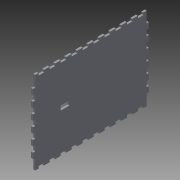
# Autodesk Inventor part: zijplaat
Saved by Autodesk Inventor 2015 (Build 190159000, 159)
## iProperties
Created: 2016-03-10
Part Number: zijplaat
Material: Generic
Document SubType Name: Modeling
Designer: david
Density: 1 g/cm^3
Appearance: Default
Author: david
Autodesk Inventor part; units mm, degrees
ref_plane "YZ Plane" through (0, 0, 0) normal (1, 0, 0) x (0, 1, 0)
ref_plane "XZ Plane" through (0, 0, 0) normal (0, 1, 0) x (-1, 0, 0)
ref_plane "XY Plane" through (0, 0, 0) normal (0, 0, 1) x (1, 0, 0)
sketch "Sketch1" plane through (0, 0, 0) normal (1, 0, 0) x (0, 1, 0)
  line L0 (0, 0) -> (210, 0)
  line L1 (210, 0) -> (210, 150)
  line L2 (210, 150) -> (0, 150)
  line L3 (0, 150) -> (0, 0)
  line L4 (66, 79) -> (50, 79)
  line L5 (50, 79) -> (50, 71)
  line L6 (50, 71) -> (66, 71)
  line L7 (66, 71) -> (66, 79)
  line L8 (0, 140) -> (4, 140)
  line L9 (4, 140) -> (4, 130)
  line L10 (4, 130) -> (0, 130)
  line L11 (0, 130) -> (0, 140)
  line L12 (0, 120) -> (4, 120)
  line L13 (4, 120) -> (4, 110)
  line L14 (4, 110) -> (0, 110)
  line L15 (0, 110) -> (0, 120)
  line L16 (0, 100) -> (4, 100)
  line L17 (4, 100) -> (4, 90)
  line L18 (4, 90) -> (0, 90)
  line L19 (0, 90) -> (0, 100)
  line L20 (0, 80) -> (4, 80)
  line L21 (4, 80) -> (4, 70)
  line L22 (4, 70) -> (0, 70)
  line L23 (0, 70) -> (0, 80)
  line L24 (0, 60) -> (4, 60)
  line L25 (4, 60) -> (4, 50)
  line L26 (4, 50) -> (0, 50)
  line L27 (0, 50) -> (0, 60)
  line L28 (0, 40) -> (4, 40)
  line L29 (4, 40) -> (4, 30)
  line L30 (4, 30) -> (0, 30)
  line L31 (0, 30) -> (0, 40)
  line L32 (0, 20) -> (4, 20)
  line L33 (4, 20) -> (4, 10)
  line L34 (4, 10) -> (0, 10)
  line L35 (0, 10) -> (0, 20)
  line L36 (10, 150) -> (20, 150)
  line L37 (20, 150) -> (20, 146)
  line L38 (20, 146) -> (10, 146)
  line L39 (10, 146) -> (10, 150)
  line L40 (30, 150) -> (40, 150)
  line L41 (40, 150) -> (40, 146)
  line L42 (40, 146) -> (30, 146)
  line L43 (30, 146) -> (30, 150)
  line L44 (50, 150) -> (60, 150)
  line L45 (60, 150) -> (60, 146)
  line L46 (60, 146) -> (50, 146)
  line L47 (50, 146) -> (50, 150)
  line L48 (70, 150) -> (80, 150)
  line L49 (80, 150) -> (80, 146)
  line L50 (80, 146) -> (70, 146)
  line L51 (70, 146) -> (70, 150)
  line L52 (90, 150) -> (100, 150)
  line L53 (100, 150) -> (100, 146)
  line L54 (100, 146) -> (90, 146)
  line L55 (90, 146) -> (90, 150)
  line L56 (110, 150) -> (120, 150)
  line L57 (120, 150) -> (120, 146)
  line L58 (120, 146) -> (110, 146)
  line L59 (110, 146) -> (110, 150)
  line L60 (130, 150) -> (140, 150)
  line L61 (140, 150) -> (140, 146)
  line L62 (140, 146) -> (130, 146)
  line L63 (130, 146) -> (130, 150)
  line L64 (150, 150) -> (160, 150)
  line L65 (160, 150) -> (160, 146)
  line L66 (160, 146) -> (150, 146)
  line L67 (150, 146) -> (150, 150)
  line L68 (170, 150) -> (180, 150)
  line L69 (180, 150) -> (180, 146)
  line L70 (180, 146) -> (170, 146)
  line L71 (170, 146) -> (170, 150)
  line L72 (190, 150) -> (200, 150)
  line L73 (200, 150) -> (200, 146)
  line L74 (200, 146) -> (190, 146)
  line L75 (190, 146) -> (190, 150)
  line L76 (0, 10) -> (4, 10)
  line L77 (4, 10) -> (4, 0)
  line L78 (4, 0) -> (0, 0)
  line L79 (0, 0) -> (0, 10)
  line L80 (0, 140) -> (4, 140)
  line L81 (4, 140) -> (4, 150)
  line L82 (4, 150) -> (0, 150)
  line L83 (0, 150) -> (0, 140)
  line L84 (10, 0) -> (20, 0)
  line L85 (20, 0) -> (20, 4)
  line L86 (20, 4) -> (10, 4)
  line L87 (10, 4) -> (10, 0)
  line L88 (30, 0) -> (40, 0)
  line L89 (40, 0) -> (40, 4)
  line L90 (40, 4) -> (30, 4)
  line L91 (30, 4) -> (30, 0)
  line L92 (50, 0) -> (60, 0)
  line L93 (60, 0) -> (60, 4)
  line L94 (60, 4) -> (50, 4)
  line L95 (50, 4) -> (50, 0)
  line L96 (70, 0) -> (80, 0)
  line L97 (80, 0) -> (80, 4)
  line L98 (80, 4) -> (70, 4)
  line L99 (70, 4) -> (70, 0)
  line L100 (90, 0) -> (100, 0)
  line L101 (100, 0) -> (100, 4)
  line L102 (100, 4) -> (90, 4)
  line L103 (90, 4) -> (90, 0)
  line L104 (110, 0) -> (120, 0)
  line L105 (120, 0) -> (120, 4)
  line L106 (120, 4) -> (110, 4)
  line L107 (110, 4) -> (110, 0)
  line L108 (130, 0) -> (140, 0)
  line L109 (140, 0) -> (140, 4)
  line L110 (140, 4) -> (130, 4)
  line L111 (130, 4) -> (130, 0)
  line L112 (150, 0) -> (160, 0)
  line L113 (160, 0) -> (160, 4)
  line L114 (160, 4) -> (150, 4)
  line L115 (150, 4) -> (150, 0)
  line L116 (170, 0) -> (180, 0)
  line L117 (180, 0) -> (180, 4)
  line L118 (180, 4) -> (170, 4)
  line L119 (170, 4) -> (170, 0)
  line L120 (190, 0) -> (200, 0)
  line L121 (200, 0) -> (200, 4)
  line L122 (200, 4) -> (190, 4)
  line L123 (190, 4) -> (190, 0)
  line L124 (210, 140) -> (206, 140)
  line L125 (206, 140) -> (206, 130)
  line L126 (206, 130) -> (210, 130)
  line L127 (210, 130) -> (210, 140)
  line L128 (210, 120) -> (206, 120)
  line L129 (206, 120) -> (206, 110)
  line L130 (206, 110) -> (210, 110)
  line L131 (210, 110) -> (210, 120)
  line L132 (210, 100) -> (206, 100)
  line L133 (206, 100) -> (206, 90)
  line L134 (206, 90) -> (210, 90)
  line L135 (210, 90) -> (210, 100)
  line L136 (210, 80) -> (206, 80)
  line L137 (206, 80) -> (206, 70)
  line L138 (206, 70) -> (210, 70)
  line L139 (210, 70) -> (210, 80)
  line L140 (210, 60) -> (206, 60)
  line L141 (206, 60) -> (206, 50)
  line L142 (206, 50) -> (210, 50)
  line L143 (210, 50) -> (210, 60)
  line L144 (210, 40) -> (206, 40)
  line L145 (206, 40) -> (206, 30)
  line L146 (206, 30) -> (210, 30)
  line L147 (210, 30) -> (210, 40)
  line L148 (210, 20) -> (206, 20)
  line L149 (206, 20) -> (206, 10)
  line L150 (206, 10) -> (210, 10)
  line L151 (210, 10) -> (210, 20)
  line L152 (206, 140) -> (206, 150)
  line L153 (206, 10) -> (206, 0)
  line L154 (206, 10) -> (210, 10)
  line L155 (210, 10) -> (210, 0)
  line L156 (210, 0) -> (206, 0)
  line L157 (206, 0) -> (206, 10)
  point P0 (0, 130)
  point P1 (0, 110)
  point P2 (0, 90)
  point P3 (0, 70)
  point P4 (0, 50)
  point P5 (0, 30)
  point P6 (24, 0)
  point P7 (44, 0)
  point P8 (64, 0)
  point P9 (84, 0)
  point P10 (104, 0)
  point P11 (124, 0)
  point P12 (144, 0)
  point P13 (164, 0)
  point P14 (184, 0)
  point P15 (210, 130)
  point P16 (210, 110)
  point P17 (210, 90)
  point P18 (210, 70)
  point P19 (210, 50)
  point P20 (210, 30)
  dimension "d0" = 150
  dimension "d1" = 210
  dimension "d2" = 8
  dimension "d3" = 16
  dimension "d4" = 71
  dimension "d5" = 50
  dimension "d6" = 4
  dimension "d7" = 10
  dimension "d8" = 10
  dimension "d11" = 20
  dimension "d16" = 4
  dimension "d17" = 10
  dimension "d18" = 10
  dimension "d21" = 20
  dimension "d26" = 4
  dimension "d27" = 10
  dimension "d30" = 20
  dimension "d35" = 4
  dimension "d36" = 10
  dimension "d37" = 10
  dimension "d40" = 20
  constraints: 316 end point, 18 parallel, 11 horizontal, 10 perpendicular, 10 point on line, 4 collinear, 2 vertical, 257 other
  measures "d0" distance of L2.end L0.start
  measures "d1" distance of L0.start L0.end
  measures "d2" distance of L6.end L4.start
  measures "d3" distance of L5.end L6.end
  measures "d4" distance between parallel lines of L4 L2
  measures "d5" distance between parallel lines of L3 L5
  measures "d6" distance between parallel lines of L3 L9
  measures "d7" distance between parallel lines of L2 L8
  measures "d8" distance between parallel lines of L10 L8
  measures "d11" distance of L2.end point (0, 130)
  measures "d16" distance between parallel lines of L36 L38
  measures "d17" distance between parallel lines of L39 L37
  measures "d18" distance between parallel lines of L3 L39
  measures "d21" distance of L38.end L42.end
  measures "d26" distance of L86.end L84.start
  measures "d27" distance between parallel lines of L3 L87
  measures "d30" distance of L86.end L90.end
  measures "d35" distance between parallel lines of L1 L125
  measures "d36" distance between parallel lines of L2 L124
  measures "d37" distance between parallel lines of L126 L124
  measures "d40" distance of L1.end point (210, 130)
extrude "Extrusion1" add sketch "Sketch1" along normal blind 3.6 contours L77 L33 L32 L3 L30 L29 L28 L26 L25 L24 L22 L21 L20 L18 L17 L16 L14 L13 L12 L10 L9 L81 L2 L39 L38 L37 L43 L42 L41 L47 L46 L45 L51 L50 L49 L55 L54 L53 L59 L58 L57 L63 L62 L61 L67 L66 L65 L71 L70 L69 L75 L74 L73 L152 L125 L126 L1 L128 L129 L130 L132 L133 L134 L136 L137 L138 L140 L141 L142 L144 L145 L146 L148 L149 L153 L0 L121 L122 L123 L117 L118 L119 L113 L114 L115 L109 L110 L111 L105 L106 L107 L101 L102 L103 L97 L98 L99 L93 L94 L95 L89 L90 L91 L85 L86 L87
body "Solid1"
